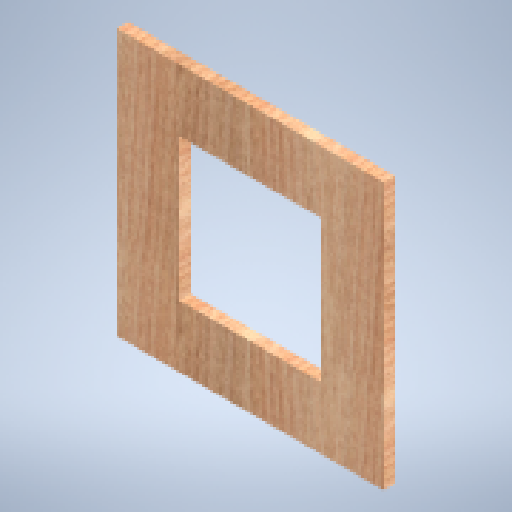
# Autodesk Inventor part: Front Plate
Saved by Autodesk Inventor 2025.1 (Build 291241000, 241)
## iProperties
Created: 2025-03-25
Part Number: Front Plate
Material: Wood (Birch)
Document SubType Name: Modeling
Designer: maxwe
Density: 0.55 g/cm^3
Appearance: Birch - Natural Polished
Author: maxwe
Autodesk Inventor part; units mm, degrees
ref_plane "YZ Plane" through (0, 0, 0) normal (1, 0, 0) x (0, 1, 0)
ref_plane "XZ Plane" through (0, 0, 0) normal (0, 1, 0) x (-1, 0, 0)
ref_plane "XY Plane" through (0, 0, 0) normal (0, 0, 1) x (1, 0, 0)
sketch "Sketch2" plane through (0, 0, 0) normal (0, 0, 1) x (1, 0, 0)
  line L0 (-150, 150) -> (150, 150)
  line L1 (150, 150) -> (150, -150)
  line L2 (150, -150) -> (-150, -150)
  line L3 (-150, -150) -> (-150, 150)
  line L4 (80, -80) -> (-80, -80)
  line L5 (-80, -80) -> (-80, 80)
  line L6 (-80, 80) -> (80, 80)
  line L7 (80, 80) -> (80, -80)
  line L8 (80, -80) -> (-80, 80) construction
  line L9 (-80, -80) -> (80, 80) construction
  point P0 (0, 0)
  point P1 (-150, 0)
  point P2 (0, 150)
  dimension "d0" = 300
  dimension "d1" = 300
  dimension "d2" = 160
  dimension "d3" = 160
  constraints: 20 end point, 4 midpoint, 4 parallel, 2 horizontal, 2 perpendicular, 1 horizontal alignment, 1 vertical alignment
  measures "d0" distance of L1.end L2.end
  measures "d1" distance of L0.end L1.end
  measures "d2" distance of L5.end L6.end
  measures "d3" distance of L4.end L5.end
extrude "Extrusion1" add sketch "Sketch2" along normal blind 12.7
body "Solid1"
